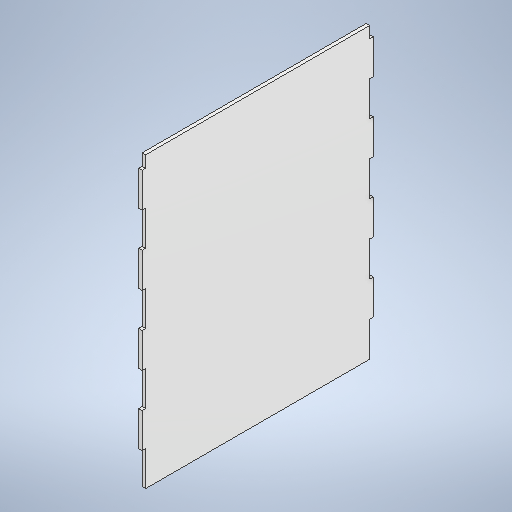
# Autodesk Inventor part: Q side 2
Saved by Autodesk Inventor 2025.3 (Build 293356000, 356)
## iProperties
Created: 2026-04-17
Part Number: Q side 2
Material: ABS Plastic
Document SubType Name: Modeling
Designer: logien
Density: 1.06 g/cm^3
Appearance: Smooth - White
Author: logien
Autodesk Inventor part; units mm, degrees
ref_plane "YZ Plane" through (0, 0, 0) normal (1, 0, 0) x (0, 1, 0)
ref_plane "XZ Plane" through (0, 0, 0) normal (0, 1, 0) x (-1, 0, 0)
ref_plane "XY Plane" through (0, 0, 0) normal (0, 0, 1) x (1, 0, 0)
sketch "Sketch2" plane through (0, 0, 0) normal (1, 0, 0) x (0, 1, 0)
  line L0 (250, 0) -> (250, -200)
  line L1 (250, -200) -> (0, -200)
  line L2 (0, -200) -> (0, 0)
  line L3 (0, 0) -> (0, -3)
  line L4 (0, -3) -> (30, -3)
  line L5 (30, -3) -> (30, 0)
  line L6 (30, 0) -> (60, 0)
  line L7 (60, 0) -> (60, -3)
  line L8 (60, -3) -> (90, -3)
  line L9 (90, -3) -> (90, 0)
  line L10 (90, 0) -> (120, 0)
  line L11 (120, 0) -> (120, -3)
  line L12 (120, -3) -> (150, -3)
  line L13 (150, -3) -> (150, 0)
  line L14 (150, 0) -> (180, 0)
  line L15 (180, 0) -> (180, -3)
  line L16 (180, -3) -> (210, -3)
  line L17 (210, -3) -> (210, 0)
  line L18 (210, 0) -> (240, 0)
  line L19 (240, 0) -> (240, -3)
  line L20 (240, -3) -> (250, -3)
  line L21 (0, -100) -> (250, -100)
  line L22 (0, -197) -> (30, -197)
  line L23 (30, -197) -> (30, -200)
  line L24 (30, -200) -> (60, -200)
  line L25 (60, -200) -> (60, -197)
  line L26 (60, -197) -> (90, -197)
  line L27 (90, -197) -> (90, -200)
  line L28 (90, -200) -> (120, -200)
  line L29 (120, -200) -> (120, -197)
  line L30 (120, -197) -> (150, -197)
  line L31 (150, -197) -> (150, -200)
  line L32 (150, -200) -> (180, -200)
  line L33 (180, -200) -> (180, -197)
  line L34 (180, -197) -> (210, -197)
  line L35 (210, -197) -> (210, -200)
  line L36 (210, -200) -> (240, -200)
  line L37 (240, -200) -> (240, -197)
  line L38 (240, -197) -> (250, -197)
  dimension "d44" = 200
  dimension "d45" = 250
  dimension "d46" = 3
  dimension "d47" = 30
  dimension "d48" = 3
  dimension "d49" = 30
  dimension "d50" = 3
  dimension "d51" = 30
  dimension "d52" = 3
  dimension "d53" = 30
  dimension "d54" = 3
  dimension "d55" = 30
  dimension "d56" = 3
  dimension "d57" = 30
  dimension "d58" = 3
  dimension "d59" = 30
  dimension "d60" = 3
  dimension "d61" = 30
  dimension "d62" = 3
  dimension "d63" = 10
  dimension "d64" = 90
  constraints: 78 end point, 18 symmetric about line, 16 point on line, 10 parallel, 2 midpoint, 1 perpendicular, 1 vertical
  measures "d44" distance of L1.end L2.end
  measures "d45" distance of L2.end L0.start
  measures "d46" distance of L2.end L3.end
  measures "d47" distance of L3.end L4.end
  measures "d48" distance of L4.end L5.end
  measures "d49" distance of L5.end L6.end
  measures "d50" distance of L6.end L7.end
  measures "d51" distance of L7.end L8.end
  measures "d52" distance of L8.end L9.end
  measures "d53" distance of L9.end L10.end
  measures "d54" distance of L10.end L11.end
  measures "d55" distance of L11.end L12.end
  measures "d56" distance of L12.end L13.end
  measures "d57" distance of L13.end L14.end
  measures "d58" distance of L14.end L15.end
  measures "d59" distance of L15.end L16.end
  measures "d60" distance of L16.end L17.end
  measures "d61" distance of L17.end L18.end
  measures "d62" distance of L18.end L19.end
  measures "d63" distance of L19.end L20.end
  measures "d64" angle of L20 L0
extrude "Extrusion2" add sketch "Sketch2" along normal blind 3 contours L0 L21 L2 L4 L5 L6 L7 L8 L9 L10 L11 L12 L13 L14 L15 L16 L17 L18 L19 L20 | L0 L38 L37 L1 L35 L34 L33 L31 L30 L29 L27 L26 L25 L23 L22 L2 L21
body "Solid2"
